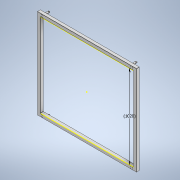
# Autodesk Inventor part: Pieza3
Saved by Autodesk Inventor 2021 (Build 250183000, 183)
## iProperties
Created: 2022-09-12
Part Number: Pieza3
Material: Genérico
Document SubType Name: Modeling
Designer: arthu
Density: 1 g/cm^3
Appearance: Valor por defecto
Author: arthu
Autodesk Inventor part; units mm, degrees
ref_plane "YZ Plane" through (0, 0, 0) normal (1, 0, 0) x (0, 1, 0)
ref_plane "XZ Plane" through (0, 0, 0) normal (0, 1, 0) x (-1, 0, 0)
ref_plane "XY Plane" through (0, 0, 0) normal (0, 0, 1) x (1, 0, 0)
sketch "Boceto1" plane through (0, 0, 0) normal (0, 0, 1) x (1, 0, 0)
  line L0 (567.5, -510) -> (-567.5, -510)
  line L1 (-567.5, -510) -> (-567.5, 510)
  line L2 (-567.5, 510) -> (567.5, 510)
  line L3 (567.5, 510) -> (567.5, -510)
  line L4 (567.5, -510) -> (-567.5, 510) construction
  line L5 (-567.5, -510) -> (567.5, 510) construction
  line L6 (605.6, 548.1) -> (-605.6, 548.1)
  line L7 (-605.6, 548.1) -> (-605.6, -548.1)
  line L8 (-605.6, -548.1) -> (605.6, -548.1)
  line L9 (605.6, -548.1) -> (605.6, 548.1)
  point P0 (0, 0)
  dimension "d0" = 1135
  dimension "d1" = 1020
  dimension "d2" = 38.1
  constraints: 20 end point, 4 parallel, 2 midpoint, 2 perpendicular, 1 horizontal, 3 other
  measures "d0" distance of L1.end L2.end
  measures "d1" distance of L0.end L1.end
  measures "d2" distance between parallel lines of L2 L6
extrude "Extrusión1" add sketch "Boceto1" along normal blind 38.1
fillet "Empalme1" radius 2 8 edges at (605.6, 548.1, 19.05) (605.6, -548.1, 19.05) (-605.6, 548.1, 19.05) (-605.6, -548.1, 19.05) (-567.5, -510, 19.05) (-567.5, 510, 19.05) (567.5, 510, 19.05) (567.5, -510, 19.05)
fillet "Empalme2" radius 2 32 edges at (-605.0142, 547.5142, 38.1) (-605.6, 0, 38.1) (-605.0142, -547.5142, 38.1) (0, -548.1, 38.1) (605.0142, -547.5142, 38.1) (605.6, 0, 38.1) (605.0142, 547.5142, 38.1) (0, 548.1, 38.1) (566.9142, 509.4142, 38.1) (567.5, 0, 38.1) (566.9142, -509.4142, 38.1) (0, -510, 38.1) (-566.9142, -509.4142, 38.1) (-567.5, 0, 38.1) (-566.9142, 509.4142, 38.1) (0, 510, 38.1) (-605.0142, 547.5142, 0) (-605.6, 0, 0) (-605.0142, -547.5142, 0) (0, -548.1, 0) (605.0142, -547.5142, 0) (605.6, 0, 0) (605.0142, 547.5142, 0) (0, 548.1, 0) (566.9142, 509.4142, 0) (567.5, 0, 0) (566.9142, -509.4142, 0) (0, -510, 0) (-566.9142, -509.4142, 0) (-567.5, 0, 0) (-566.9142, 509.4142, 0) (0, 510, 0)
sketch "Boceto2" plane through (0, 0, 0) normal (0, 0, -1) x (-1, 0, 0)
  line L0 (-603.6, 546.1) -> (-603.6, -546.1) projected
  line L1 (-603.6, 546.1) -> (-543.6, 546.1)
  line L2 (603.6, 546.1) -> (-603.6, 546.1) projected
  line L3 (-603.6, 548.1) -> (603.6, 548.1) projected
  line L4 (-543.6, 548.1) -> (-547.6, 548.1)
  line L5 (-543.6, 548.1) -> (-543.6, 544.1)
  line L6 (-543.6, 544.1) -> (-521.6, 544.1)
  line L7 (-521.6, 544.1) -> (-521.6, 548.1)
  line L8 (-521.6, 548.1) -> (-543.6, 548.1)
  line L9 (-543.6, 548.1) -> (-543.6, 544.1)
  line L10 (0, 548.1) -> (0, -512)
  line L11 (565.5, -512) -> (-565.5, -512) projected
  line L12 (-565.5, 0) -> (567.5, 0)
  line L13 (567.5, -508) -> (567.5, 508) projected
  line L14 (-603.6, -548.1) -> (603.6, -548.1)
  line L15 (-543.6, -548.1) -> (-543.6, -544.1)
  line L16 (-543.6, -544.1) -> (-521.6, -544.1)
  line L17 (-521.6, -544.1) -> (-521.6, -548.1)
  line L18 (543.6, 548.1) -> (543.6, 544.1)
  line L19 (543.6, 544.1) -> (521.6, 544.1)
  line L20 (521.6, 544.1) -> (521.6, 548.1)
  line L21 (521.6, 548.1) -> (543.6, 548.1)
  line L22 (543.6, -544.1) -> (521.6, -544.1)
  line L23 (521.6, -544.1) -> (521.6, -548.1)
  line L24 (603.6, -548.1) -> (-603.6, -548.1)
  line L25 (543.6, -548.1) -> (543.6, -544.1)
  point P0 (0, 0)
  point P1 (543.6, 546.1)
  dimension "d7" = 60
  dimension "d8" = 4
  dimension "d9" = 4
  dimension "d10" = 22
  constraints: 42 end point, 18 symmetric about line, 8 point on line, 3 midpoint, 2 parallel, 1 horizontal, 1 perpendicular, 1 vertical
  measures "d7" distance of L0.start L1.end
  measures "d8" distance of L4.start L4.end
  measures "d9" distance of L4.start L5.end
  measures "d10" distance of L8.end L7.end
extrude "Extrusión2" add sketch "Boceto2" along normal blind 40 contours L18 L19 L20 L2 | L2 L20 L3 L18 | L7 L6 L5 L2 | L2 L5 L3 L7 | L15 L16 L17 L14 | L23 L22 L25 L14
fillet "Empalme3" radius 10 8 edges at (543.6, -546.1, -40) (521.6, -546.1, -40) (543.6, 546.1, -40) (521.6, 546.1, -40) (-521.6, 546.1, -40) (-543.6, 546.1, -40) (-543.6, -546.1, -40) (-521.6, -546.1, -40)
sketch "Boceto3" plane through (521.6, -548.1, 0) normal (0, -1, 0) x (1, 0, 0)
  line L0 (22, 0) -> (0, 0) projected
  line L1 (0, 0) -> (22, 0)
  line L2 (22, 0) -> (22, -40)
  line L3 (22, -40) -> (0, -40)
  line L4 (0, -40) -> (0, 0)
  circle A0 centre (11, -29) radius 11
  circle A1 centre (11, -29) radius 5
  point P0 (-521.6, 0)
  dimension "d14" = 10
  constraints: 8 end point, 3 tangent, 2 centre point, 2 parallel, 1 coincident, 1 horizontal, 1 perpendicular
  measures "d14" diameter of A1
extrude "Extrusión3" cut sketch "Boceto3" against normal blind 20000 contours A1
sketch "Boceto4" plane through (-543.6, -548.1, 0) normal (0, -1, 0) x (1, 0, 0)
  line L0 (0, 0) -> (0, -30) projected
  line L1 (0, 0) -> (22, 0)
  line L2 (22, 0) -> (22, -40)
  line L3 (22, -40) -> (0, -40)
  line L4 (0, -40) -> (0, 0)
  circle A0 centre (11, -29) radius 11
  circle A1 centre (11, -29) radius 5
  point P0 (543.6, 0)
  dimension "d17" = 10
  constraints: 8 end point, 3 tangent, 2 centre point, 2 parallel, 1 coincident, 1 horizontal, 1 perpendicular
  measures "d17" diameter of A1
extrude "Extrusión4" cut sketch "Boceto4" against normal blind 20000 contours A1
sketch "Boceto5" plane through (0, 0, 38.1) normal (0, 0, 1) x (1, 0, 0)
  line L0 (-565.5, 510) -> (565.5, 510) projected
  line L1 (565.5, -510) -> (-565.5, -510) projected
  point P0 (0, 0)
  dimension "d20" = 1020
  measures "d20" distance between parallel lines of L0 L1
sketch "Boceto6" plane through (0, 0, 38.1) normal (0, 0, 1) x (1, 0, 0)
  line L0 (565.5, -510) -> (-565.5, -510) projected
  line L1 (543.6, -548.1) -> (521.6, -548.1) projected
  line L2 (565.5, -510) -> (527.4, -510)
  line L3 (527.4, -510) -> (527.4, -548.1)
  line L4 (527.4, -548.1) -> (565.5, -548.1)
  line L5 (565.5, -548.1) -> (565.5, -510)
  line L6 (555.5, -538.1) -> (537.4, -538.1)
  line L7 (537.4, -538.1) -> (537.4, -520)
  line L8 (537.4, -520) -> (555.5, -520)
  line L9 (555.5, -520) -> (555.5, -538.1)
  circle A0 centre (555.5, -538.1) radius 2.5
  circle A1 centre (555.5, -520) radius 2.5
  circle A2 centre (537.4, -538.1) radius 2.5
  circle A3 centre (537.4, -520) radius 2.5
  line L10 (0, 0) -> (0, -570.6664)
  line L11 (0, 0) -> (796.3032, 0)
  line L12 (-565.5, -510) -> (-527.4, -510)
  line L13 (-527.4, -510) -> (-527.4, -548.1)
  line L14 (-527.4, -548.1) -> (-565.5, -548.1)
  line L15 (-565.5, -548.1) -> (-565.5, -510)
  circle A4 centre (-555.5, -538.1) radius 2.5
  circle A5 centre (-555.5, -520) radius 2.5
  circle A6 centre (-537.4, -538.1) radius 2.5
  circle A7 centre (-537.4, -520) radius 2.5
  line L16 (565.5, 510) -> (-565.5, 510)
  line L17 (527.4, 510) -> (527.4, 548.1)
  line L18 (527.4, 548.1) -> (565.5, 548.1)
  line L19 (565.5, 548.1) -> (565.5, 510)
  circle A8 centre (555.5, 538.1) radius 2.5
  circle A9 centre (555.5, 520) radius 2.5
  circle A10 centre (537.4, 538.1) radius 2.5
  circle A11 centre (537.4, 520) radius 2.5
  line L20 (-527.4, 510) -> (-527.4, 548.1)
  line L21 (-527.4, 548.1) -> (-565.5, 548.1)
  line L22 (-565.5, 548.1) -> (-565.5, 510)
  circle A12 centre (-555.5, 538.1) radius 2.5
  circle A13 centre (-537.4, 538.1) radius 2.5
  circle A14 centre (-537.4, 520) radius 2.5
  circle A15 centre (-555.5, 520) radius 2.5
  line L23 (-565.5, 510) -> (-527.4, 510)
  dimension "d21" = 38.1
  dimension "d22" = 10
  dimension "d23" = 5
  dimension "d24" = 5
  dimension "d25" = 5
  dimension "d26" = 5
  constraints: 44 end point, 23 symmetric about line, 16 centre point, 4 coincident, 4 parallel, 2 horizontal, 2 perpendicular, 1 point on line, 1 vertical, 15 other
  measures "d21" distance of L4.end L3.end
  measures "d22" distance between parallel lines of L4 L6
  measures "d23" diameter of A0
  measures "d24" diameter of A1
  measures "d25" diameter of A2
  measures "d26" diameter of A3
extrude "Extrusión5" cut sketch "Boceto6" against normal blind 5 contours A2 L7 L6 | L6 L7 A2 | A0 L9 L6 | L6 L9 A0 | A3 L8 L7 | L7 L8 A3 | A1 L8 L9 | L9 L8 A1 | A4 | A5 | A6 | A7 | A8 | A9 | A10 | A11 | A12 | A13 | A14 | A15
equation "\"d27\" = d24"
